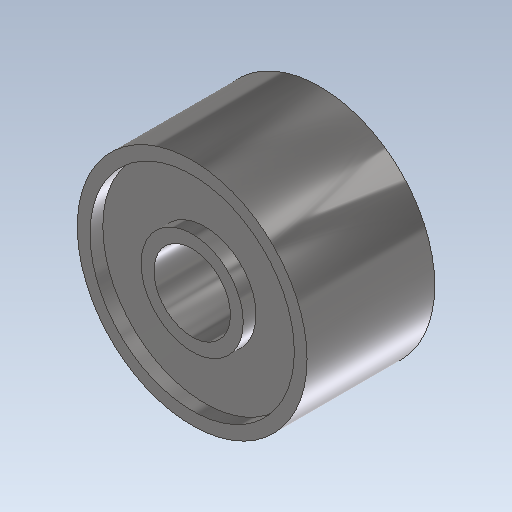
# Autodesk Inventor part: ベアリングd3D9B5F無
Saved by Autodesk Inventor 2020.2 (Build 242310000, 310)
## iProperties
Created: 2017-02-12
Part Number: ベアリングd3D9B5F無
Material: 鋼、炭素鋼
Document SubType Name: Modeling
Designer: 大空
Mass: 0.77 g
Surface Area: 3.39292 cm^2
Volume: 0.245044 cm^3
Density: 3.14229 g/cm^3
Appearance: 半つや出し
Author: 大空
Autodesk Inventor part; units mm, degrees
ref_plane "YZ Plane" through (0, 0, 0) normal (1, 0, 0) x (0, 1, 0)
ref_plane "XZ Plane" through (0, 0, 0) normal (0, 1, 0) x (-1, 0, 0)
ref_plane "XY Plane" through (0, 0, 0) normal (0, 0, 1) x (1, 0, 0)
sketch "スケッチ1" plane through (0, 0, 0) normal (0, 0, 1) x (1, 0, 0)
  circle A0 centre (0, 0) radius 1.5
  circle A1 centre (0, 0) radius 4.5
  dimension "d0" = 3
  dimension "d1" = 9
  constraints: 2 centre point, 2 coincident
  measures "d0" diameter of A0
  measures "d1" diameter of A1
extrude "押し出し1" add sketch "スケッチ1" along normal blind 5
sketch "スケッチ3" plane through (0, 0, 5) normal (0, 0, 1) x (1, 0, 0)
  circle A0 centre (0, 0) radius 1.5 projected
  circle A1 centre (0, 0) radius 4.5 projected
  circle A2 centre (0, 0) radius 4
  circle A3 centre (0, 0) radius 2
  dimension "d7" = 0.5
  dimension "d8" = 0.5
  constraints: 2 centre point
  measures "d7" radial gap between concentric circles of A1 A2
  measures "d8" radial gap between concentric circles of A0 A3
extrude "押し出し3" cut sketch "スケッチ3" against normal blind 0.5 contours A2
sketch "スケッチ7" plane through (0, 0, 0) normal (0, 0, -1) x (-1, 0, 0)
  circle A0 centre (0, 0) radius 2 projected
  circle A1 centre (0, 0) radius 4 projected
extrude "押し出し6" cut sketch "スケッチ7" against normal blind 0.5
